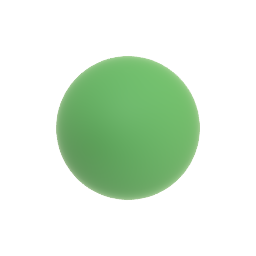
Assembly (Autodesk Fusion 360 archive; units mm, degrees)
design "Ball"
Autodesk Fusion 360 part; units mm, degrees
sphere "SpherePrimitive1" add diameter 40 placed x (1, 0, 0) y (0, 1, 0) z (0, 0, 1) at (0, 0, 0) makes body 1 in component "Ball"
sketch "Sketch1" plane through (0, 0, 0) normal (0, 0, 1) x (1, 0, 0) in component "Ramp"
  line L0 (-60, 30) -> (60, 30)
  line L1 (60, 30) -> (60, -30)
  line L2 (60, -30) -> (-60, -30)
  line L3 (-60, -30) -> (-60, 30)
  line L4 (-60, 30) -> (60, -30) construction
  line L5 (60, 30) -> (-60, -30) construction
  dimension "d2" = 120
  dimension "d3" = 60
  constraint horizontal L0
  constraint perpendicular L0 L1
  constraint parallel L0 L2
  constraint parallel L1 L3
  constraint coincident L4 origin
  constraint coincident L5 origin
  measures "d2" distance of L1.end L2.end
  measures "d3" distance of L0.end L1.end
extrude "Extrude1" add sketch "Sketch1" along normal blind 50 separate body makes body 2 in component "Ramp"
sketch "Sketch2" plane through (-60, 0, 0) normal (-1, 0, 0) x (0, -1, 0) in component "Ramp"
  line L0 (-30, 0) -> (30, 0)
  line L1 (30, 0) -> (30, 50)
  line L2 (30, 50) -> (-30, 50)
  line L3 (-30, 50) -> (-30, 0)
  circle A0 centre (0, 50) radius 25
  dimension "d6" = 50
  constraint midpoint L2 A0.centre
  measures "d6" diameter of A0
extrude "Extrude2" cut sketch "Sketch2" against normal blind 140 contours L2 A0 picked at (-4.1667, 42.7831) bodies 2 in component "Ramp"
extrude "Extrude3" add 1 faces at (20, -10, 0) along direction (0, 0, -1) blind 10 on bodies 2 bodies 2 in component "Ramp"
sketch "Sketch3" plane through (60, 0, 0) normal (1, 0, 0) x (0, 1, 0) in component "Ramp"
  arc A0 (-25, 50) -> (25, 50) centre (0, 50) ccw
  line L0 (-25, 50) -> (-30, 50)
  line L1 (-30, 50) -> (-30, -10)
  line L2 (-30, -10) -> (30, -10)
  line L3 (30, -10) -> (30, 50)
  line L4 (30, 50) -> (25, 50)
  circle A1 centre (-30, 50) radius 60
  circle A2 centre (30, 50) radius 60
  constraint coincident L0.end L1.start
  constraint coincident L3.end A1
  constraint coincident L3.end L4.start
  constraint coincident L0.end A2
extrude "Extrude4" cut sketch "Sketch3" against normal blind 165 contours L1 A1 A2 | L3 A1 A2 | L2 A1 A2 picked at (-21.1858, 5.1301) picked at (21.1858, 5.1301) bodies 2 in component "Ramp"
fillet "Fillet1" radius 15 1 edges at (0, 0, -1.9615) on bodies 2 in component "Ramp"
fillet "Fillet2" radius 2.5 4 edges at (0, -30, 50) (0, -25, 50) (0, 25, 50) (0, 30, 50) on bodies 2 in component "Ramp"
move_body "MoveFace1" bodies 1 to x (1, 0, 0) y (0, 1, 0) z (0, 0, 1) at (0, 0, 46) on bodies 1 in component "Ball"
component "Ball" placed x (1, 0, 0) y (0, 1, 0) z (0, 0, 1) at (0, 0, 0)

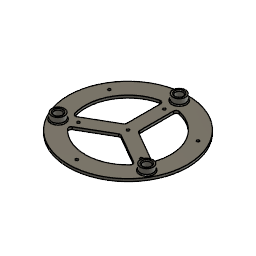
design "Tri table top"
Autodesk Fusion 360 part; units mm, degrees
sketch "Sketch1" plane through (0, 0, 0) normal (0, 1, 0) x (1, 0, 0)
  circle A0 centre (0, 0) radius 70
  dimension "d1" = 140
  constraint coincident A0.centre origin
  measures "d1" diameter of A0
extrude "Extrude1" add sketch "Sketch1" along normal blind 3
sketch "Sketch2" plane through (0, 3, 0) normal (0, 1, 0) x (-1, 0, 0)
  circle A0 centre (0, 0) radius 70
  line L0 (0, -70) -> (0, 70) construction
  line L1 (70, 0) -> (-70, 0) construction
  circle A1 centre (0, 0) radius 60 construction
  circle A2 centre (0, -60) radius 4.575
  circle A3 centre (0, -60) radius 7.5
  circle A4 centre (0, 60) radius 1.5
  dimension "d4" = 120
  dimension "d5" = 9.15
  dimension "d6" = 15
  dimension "d16" = 3
  constraint coincident A0 L0.start
  constraint coincident A0 L0.end
  constraint vertical L0
  constraint coincident A0 L1.start
  constraint coincident A0 L1.end
  constraint horizontal L1
  constraint concentric A0 A1
  constraint coincident A1 A2.centre
  constraint coincident L0 A2.centre
  constraint concentric A2 A3
  constraint coincident A1 A4.centre
  constraint coincident L0 A4.centre
  measures "d4" diameter of A1
  measures "d5" diameter of A2
  measures "d6" diameter of A3
  measures "d16" diameter of A4
extrude "Extrude2" add sketch "Sketch2" along normal blind 7 contours A3
sketch "Sketch3" plane through (0, 3, 0) normal (0, 1, 0) x (-1, 0, 0)
  circle A0 centre (0, -60) radius 4.575
  circle A1 centre (0, -60) radius 1.5
  dimension "d9" = 3
  constraint concentric A0 A1
  measures "d9" diameter of A1
extrude "Extrude3" cut sketch "Sketch3" against normal blind 25 contours A1
pattern_circular "C-Pattern1" count 3 over 360 about axis through (0, 1.75, 0) along (0, 1, 0) of "Extrude2"
pattern_circular "C-Pattern2" count 3 over 360 about axis through (0, 1.75, 0) along (0, 1, 0) of "Extrude3"
extrude "Extrude4" cut sketch "Sketch2" against normal blind 19 contours A4
pattern_circular "C-Pattern3" count 3 over 360 about axis through (0, 1.75, 0) along (0, 1, 0) of "Extrude4"
sketch "Sketch4" plane through (0, 3, 0) normal (0, 1, 0) x (-1, 0, 0)
  circle A0 centre (51.9615, -30) radius 1.5
  circle A1 centre (-51.9615, -30) radius 1.5
  circle A2 centre (0, 60) radius 1.5
  circle A3 centre (51.9615, 30) radius 7.5
  circle A4 centre (0, 0) radius 70
  circle A5 centre (0, -60) radius 7.5
  circle A6 centre (-51.9615, 30) radius 7.5
  circle A7 centre (0, 0) radius 7.5
  circle A8 centre (0, 0) radius 50
  line L0 (7.5, -50.9302) -> (-7.5, -50.9302)
  line L1 (-7.5, -50.9302) -> (-7.5, -2.3436)
  line L2 (-7.5, -2.3436) -> (7.5, -2.3436)
  line L3 (7.5, -2.3436) -> (7.5, -50.9302)
  line L4 (7.5, -50.9302) -> (-7.5, -2.3436) construction
  line L5 (-7.5, -50.9302) -> (7.5, -2.3436) construction
  line L6 (-1.7204, 7.667) -> (40.3568, 31.9603)
  line L7 (47.8568, 18.9699) -> (5.7796, -5.3234)
  line L8 (-5.7796, -5.3234) -> (-47.8568, 18.9699)
  line L9 (-40.3568, 31.9603) -> (1.7204, 7.667)
  point P0 (0, -26.6369)
  dimension "d21" = 15
  dimension "d22" = 100
  dimension "d23" = 15
  dimension "d25" = 360
  constraint concentric A4 A7
  constraint concentric A4 A8
  constraint horizontal L0
  constraint perpendicular L0 L1
  constraint parallel L0 L2
  constraint parallel L1 L3
  constraint coincident L4 P0
  constraint coincident L5 P0
  measures "d21" diameter of A7
  measures "d22" diameter of A8
  measures "d23" distance of L1.end L2.end
extrude "Extrude5" cut sketch "Sketch4" against normal blind 7 contours A8 L1 L8 | A8 L3 L7 | A8 L6 L9
sketch "Sketch5" plane through (0, 3, 0) normal (0, 1, 0) x (-1, 0, 0)
  line L0 (7.5, -4.3301) -> (46.5614, 18.222)
  arc A0 (7.5, -49.4343) -> (46.5614, 18.222) centre (0, 0) ccw
  line L1 (7.5, -49.4343) -> (7.5, -4.3301)
  line L2 (-46.5614, 18.222) -> (-7.5, -4.3301)
  line L3 (-7.5, -4.3301) -> (-7.5, -49.4343)
  arc A1 (-46.5614, 18.222) -> (-7.5, -49.4343) centre (0, 0) ccw
  line L4 (0, 8.6603) -> (-39.0614, 31.2123)
  arc A2 (39.0614, 31.2123) -> (-39.0614, 31.2123) centre (0, 0) ccw
  line L5 (39.0614, 31.2123) -> (0, 8.6603)
  circle A3 centre (51.9615, -30) radius 1.5
  circle A4 centre (-51.9615, -30) radius 1.5
  circle A5 centre (0, 60) radius 1.5
  circle A6 centre (51.9615, 30) radius 7.5
  circle A7 centre (0, 0) radius 70
  circle A8 centre (0, -60) radius 7.5
  circle A9 centre (-51.9615, 30) radius 7.5
  circle A10 centre (0, 0) radius 42.5 construction
  circle A11 centre (0, -42.5) radius 1.5
  dimension "d28" = 85
  dimension "d29" = 3
  constraint concentric A0 A10
  constraint coincident A10 A11.centre
  measures "d28" diameter of A10
  measures "d29" diameter of A11
extrude "Extrude6" cut sketch "Sketch5" against normal blind 16 contours A11
pattern_circular "C-Pattern4" count 3 over 360 about axis through (0, 1.75, 0) along (0, 1, 0) of "Extrude6"
fillet "Fillet1" radius 3 6 edges at (-7.5, 1.5, -49.4343) (7.5, 1.5, -49.4343) (-46.5614, 1.5, 18.222) (-39.0614, 1.5, 31.2123) (39.0614, 1.5, 31.2123) (46.5614, 1.5, 18.222)
sketch "Sketch6" plane through (0, 3, 0) normal (0, 1, 0) x (-1, 0, 0)
  circle A0 centre (-36.8061, 21.25) radius 1.5
  circle A1 centre (36.8061, 21.25) radius 1.5
  circle A2 centre (0, -42.5) radius 1.5
  line L0 (7.5, -4.3301) -> (43.4245, 16.4109)
  arc A3 (47.792, 14.6945) -> (43.4245, 16.4109) centre (44.9245, 13.8128) ccw
  arc A4 (11.1702, -48.7363) -> (47.792, 14.6945) centre (0, 0) ccw
  arc A5 (7.5, -45.8121) -> (11.1702, -48.7363) centre (10.5, -45.8121) ccw
  line L1 (7.5, -45.8121) -> (7.5, -4.3301)
  line L2 (-43.4245, 16.4109) -> (-7.5, -4.3301)
  line L3 (-7.5, -4.3301) -> (-7.5, -45.8121)
  arc A6 (-11.1702, -48.7363) -> (-7.5, -45.8121) centre (-10.5, -45.8121) ccw
  arc A7 (-47.792, 14.6945) -> (-11.1702, -48.7363) centre (0, 0) ccw
  arc A8 (-43.4245, 16.4109) -> (-47.792, 14.6945) centre (-44.9245, 13.8128) ccw
  line L4 (0, 8.6603) -> (-35.9245, 29.4012)
  arc A9 (-36.6218, 34.0418) -> (-35.9245, 29.4012) centre (-34.4245, 31.9993) ccw
  arc A10 (36.6218, 34.0418) -> (-36.6218, 34.0418) centre (0, 0) ccw
  arc A11 (35.9245, 29.4012) -> (36.6218, 34.0418) centre (34.4245, 31.9993) ccw
  line L5 (35.9245, 29.4012) -> (0, 8.6603)
  circle A12 centre (51.9615, -30) radius 1.5
  circle A13 centre (-51.9615, -30) radius 1.5
  circle A14 centre (0, 60) radius 1.5
  circle A15 centre (51.9615, 30) radius 7.5
  circle A16 centre (0, 0) radius 70
  circle A17 centre (0, -60) radius 7.5
  circle A18 centre (-51.9615, 30) radius 7.5
  circle A19 centre (0, 0) radius 1.5
  dimension "d36" = 3
  constraint coincident A4.centre A7.centre
  measures "d36" diameter of A19
extrude "Extrude7" cut sketch "Sketch6" against normal blind 12 contours A19
fillet "Fillet2" radius 3 3 edges at (-7.5, 1.5, -4.3301) (7.5, 1.5, -4.3301) (0, 1.5, 8.6603)
fillet "Fillet3" radius 1 3 edges at (-53.109, 3, 22.5883) (46.1165, 3, 34.6996) (6.9925, 3, -57.2879)
chamfer "Chamfer1" distance 1 angle 45 3 edges at (4.2654, 10, -58.3456) (48.3961, 10, 32.8667) (-52.6615, 10, 25.4789)

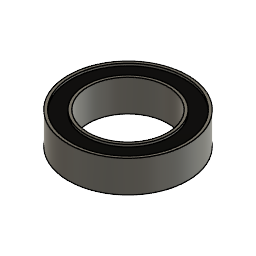
design "Bearing 15 x 10 x 4"
Autodesk Fusion 360 part; units mm, degrees
sketch "Sketch1" plane through (0, 0, 0) normal (0, 1, 0) x (1, 0, 0)
  circle A0 centre (0, 0) radius 7.5
  circle A1 centre (0, 0) radius 5
  dimension "d1" = 15
  dimension "d2" = 10
  constraint coincident A0.centre A1.centre
  constraint concentric A0 A1
  measures "d1" diameter of A0
  measures "d2" diameter of A1
extrude "Extrude1" add sketch "Sketch1" along normal blind 4
sketch "Sketch2" plane through (0, 4, 0) normal (0, 1, 0) x (-1, 0, 0)
  circle A0 centre (0, 0) radius 5
  circle A1 centre (0, 0) radius 7.5
  circle A2 centre (0, 0) radius 5.35
  circle A3 centre (0, 0) radius 7.15
  dimension "d5" = 10.7
  dimension "d6" = 14.3
  constraint coincident A0.centre A1.centre
  measures "d5" diameter of A2
  measures "d6" diameter of A3
sketch "Sketch3" plane through (0, 0, 0) normal (0, -1, 0) x (1, 0, 0)
  circle A0 centre (0, 0) radius 5
  circle A1 centre (0, 0) radius 7.5
  circle A2 centre (0, 0) radius 5.35
  circle A3 centre (0, 0) radius 7.15
  dimension "d7" = 10.7
  dimension "d8" = 14.3
  constraint concentric A0 A2
  constraint concentric A2 A3
  measures "d7" diameter of A2
  measures "d8" diameter of A3
extrude "Extrude2" cut sketch "Sketch3" against normal blind 0.3 contours A3
extrude "Extrude3" cut sketch "Sketch2" against normal blind 0.3 contours A3
sketch "Sketch4" plane through (0, 0, 0) normal (0, 1, 0) x (1, 0, 0)

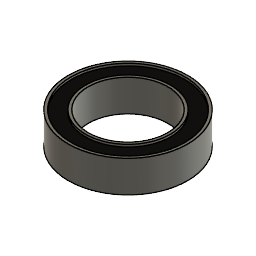
design "Bearing 15 x 10 x 4"
Autodesk Fusion 360 part; units mm, degrees
sketch "Sketch1" plane through (0, 0, 0) normal (0, 1, 0) x (1, 0, 0)
  circle A0 centre (0, 0) radius 7.5
  circle A1 centre (0, 0) radius 5
  dimension "d1" = 15
  dimension "d2" = 10
  constraint coincident A0.centre A1.centre
  constraint concentric A0 A1
  measures "d1" diameter of A0
  measures "d2" diameter of A1
extrude "Extrude1" add sketch "Sketch1" along normal blind 4
sketch "Sketch2" plane through (0, 4, 0) normal (0, 1, 0) x (-1, 0, 0)
  circle A0 centre (0, 0) radius 5
  circle A1 centre (0, 0) radius 7.5
  circle A2 centre (0, 0) radius 5.35
  circle A3 centre (0, 0) radius 7.15
  dimension "d5" = 10.7
  dimension "d6" = 14.3
  constraint coincident A0.centre A1.centre
  measures "d5" diameter of A2
  measures "d6" diameter of A3
sketch "Sketch3" plane through (0, 0, 0) normal (0, -1, 0) x (1, 0, 0)
  circle A0 centre (0, 0) radius 5
  circle A1 centre (0, 0) radius 7.5
  circle A2 centre (0, 0) radius 5.35
  circle A3 centre (0, 0) radius 7.15
  dimension "d7" = 10.7
  dimension "d8" = 14.3
  constraint concentric A0 A2
  constraint concentric A2 A3
  measures "d7" diameter of A2
  measures "d8" diameter of A3
extrude "Extrude2" cut sketch "Sketch3" against normal blind 0.3 contours A3
extrude "Extrude3" cut sketch "Sketch2" against normal blind 0.3 contours A3
sketch "Sketch4" plane through (0, 0, 0) normal (0, 1, 0) x (1, 0, 0)
